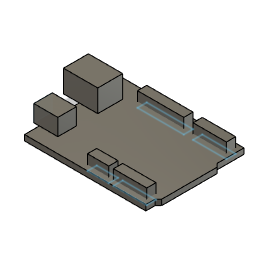
Arduino v3 (Autodesk Fusion 360 design; units mm, degrees)
Autodesk Fusion 360 part; units mm, degrees
sketch "Sketch1" plane through (0, 0, 0) normal (0, 1, 0) x (1, 0, 0)
  line L0 (0, 0) -> (65.5, 0)
  line L1 (65.5, 0) -> (65.5, -53)
  line L2 (65.5, -53) -> (0, -53)
  line L3 (0, -53) -> (0, 0)
  line L4 (65.5, -53) -> (65.5, -48) construction
  line L5 (65.5, -48) -> (67.2678, -46.2322)
  line L6 (65.5, -48) -> (68, -48) construction
  line L7 (67.2678, -46.2322) -> (67.2678, -16.2322)
  line L8 (67.2678, -16.2322) -> (65.5, -14.4645)
  line L9 (67.2678, -16.2322) -> (64.7678, -16.2322) construction
  dimension "d1" = 65.5
  dimension "d2" = 53
  dimension "d3" = 5
  dimension "d4" = 45
  dimension "d5" = 2.5
  dimension "d6" = 30
  dimension "d7" = 45
  dimension "d8" = 2.5
  constraint horizontal L0
  constraint vertical L1
  constraint horizontal L2
  constraint vertical L3
  constraint coincident L0.start L3.end
  constraint perpendicular L2 L4
  constraint horizontal L6
  constraint perpendicular L6 L7
  constraint horizontal L9
  measures "d1" distance of L0.start L0.end
  measures "d2" distance of L0.start L2.end
  measures "d3" distance of L1.end L4.end
  measures "d4" angle of L5 L6
  measures "d5" distance of L4.end L5.end
  measures "d6" distance of L5.end L7.end
  measures "d7" angle of L8 L9
  measures "d8" distance of L7.end L8.end
sketch "Sketch2" plane through (0, 0, 0) normal (0, 1, 0) x (1, 0, 0)
  line L0 (63, -2) -> (45, -2)
  line L1 (45, -2) -> (45, -7)
  line L2 (45, -7) -> (63, -7)
  line L3 (63, -7) -> (63, -2)
  line L4 (40, -2) -> (15, -2)
  line L5 (15, -2) -> (15, -7)
  line L6 (15, -7) -> (40, -7)
  line L7 (40, -7) -> (40, -2)
  line L8 (63, -50) -> (45, -50)
  line L9 (45, -50) -> (45, -45)
  line L10 (45, -45) -> (63, -45)
  line L11 (63, -45) -> (63, -50)
  line L12 (42.5, -45) -> (31, -45)
  line L13 (31, -45) -> (31, -50)
  line L14 (31, -50) -> (42.5, -50)
  line L15 (42.5, -50) -> (42.5, -45)
  constraint horizontal L0
  constraint vertical L1
  constraint horizontal L2
  constraint vertical L3
  constraint horizontal L4
  constraint vertical L5
  constraint horizontal L6
  constraint vertical L7
  constraint horizontal L8
  constraint vertical L9
  constraint horizontal L10
  constraint vertical L11
  constraint horizontal L12
  constraint vertical L13
  constraint horizontal L14
  constraint vertical L15
extrude "Extrude1" add sketch "Sketch1" sketch "Sketch2" along normal blind 3 of sketch 2 contours L0 L1 L2 L3 | L4 L5 L6 L7 makes body 1
sketch "Sketch3" plane through (0, 0, 0) normal (0, -1, 0) x (1, 0, 0)
  line L0 (67.2678, 46.2322) -> (65.5, 48)
  line L1 (65.5, 48) -> (65.5, 53)
  line L2 (65.5, 53) -> (0, 53)
  line L3 (0, 53) -> (0, 0)
  line L4 (0, 0) -> (65.5, 0)
  line L5 (65.5, 0) -> (65.5, 14.4645)
  line L6 (65.5, 14.4645) -> (67.2678, 16.2322)
  line L7 (67.2678, 16.2322) -> (67.2678, 46.2322)
extrude "Extrude2" add sketch "Sketch2" along normal blind 8 separate body makes body 2 at (51, 2.6667, 7) makes body 3 at (34.8333, 2.6667, 50) makes body 4 at (23.3333, 2.6667, 7) makes body 5 at (57, 2.6667, 50)
sketch "Sketch4" plane through (0, 3, 0) normal (0, 1, 0) x (-1, 0, 0)
  line L0 (-65.5, 48) -> (-67.2678, 46.2322)
  line L1 (-67.2678, 46.2322) -> (-67.2678, 16.2322)
  line L2 (-67.2678, 16.2322) -> (-65.5, 14.4645)
  line L3 (-65.5, 14.4645) -> (-65.5, 0)
  line L4 (-65.5, 0) -> (0, 0)
  line L5 (0, 0) -> (0, 53)
  line L6 (0, 53) -> (-65.5, 53)
  line L7 (-65.5, 53) -> (-65.5, 48)
  line L8 (0, 35) -> (-10, 35)
  line L9 (-10, 35) -> (-10, 45)
  line L10 (-10, 45) -> (0, 45)
  line L11 (0, 45) -> (0, 35)
  line L12 (0, 35) -> (3, 35)
  line L13 (3, 35) -> (3, 45)
  line L14 (3, 45) -> (0, 45)
  line L15 (0, 45) -> (0, 35)
  constraint horizontal L8
  constraint vertical L9
  constraint horizontal L10
  constraint vertical L11
  constraint coincident L5 L8.start
  constraint horizontal L12
  constraint vertical L13
  constraint horizontal L14
  constraint vertical L15
extrude "Extrude3" add sketch "Sketch4" along normal blind 9 contours L5 L11 L12 L13 L14 L15 | L5 L8 L9 L10 L11 L15 bodies 1
sketch "Sketch5" plane through (-3, 0, 0) normal (-1, 0, 0) x (0, 0, 1)
  line L0 (35, 3) -> (45, 3)
  line L1 (45, 3) -> (45, 12)
  line L2 (45, 12) -> (35, 12)
  line L3 (35, 12) -> (35, 3)
hole "Hole1" at (-3, 7.5, 40) direction (1, 0, 0) diameter 8 depth 10 tip angle 118 bodies 1
sketch "Sketch6" plane through (-3, 7.5, 40) normal (-1, 0, 0) x (0, 0, 1)
  circle A0 centre (0, 0) radius 1
  constraint coincident A0.centre origin
extrude "Extrude4" add sketch "Sketch6" against normal blind 11 separate body makes body 6
sketch "Sketch7" plane through (0, 3, 0) normal (0, 1, 0) x (-1, 0, 0)
  line L0 (-10, 45) -> (0, 45)
  line L1 (0, 45) -> (0, 53)
  line L2 (0, 53) -> (-65.5, 53)
  line L3 (-65.5, 53) -> (-65.5, 48)
  line L4 (-65.5, 48) -> (-67.2678, 46.2322)
  line L5 (-67.2678, 46.2322) -> (-67.2678, 16.2322)
  line L6 (-67.2678, 16.2322) -> (-65.5, 14.4645)
  line L7 (-65.5, 14.4645) -> (-65.5, 0)
  line L8 (-65.5, 0) -> (0, 0)
  line L9 (0, 0) -> (0, 35)
  line L10 (0, 35) -> (-10, 35)
  line L11 (-10, 35) -> (-10, 45)
  line L12 (-10, 10) -> (8.5084, 10)
  line L13 (8.5084, 10) -> (8.5084, 23.4625)
  line L14 (8.5084, 23.4625) -> (-10, 23.4625)
  line L15 (-10, 23.4625) -> (-10, 10)
  constraint horizontal L12
  constraint vertical L13
  constraint horizontal L14
  constraint vertical L15
extrude "Extrude5" add sketch "Sketch7" along normal blind 12 contours L9 L12 L13 L14 | L9 L12 L14 L15 bodies 1
sketch "Sketch8" plane through (-8.5084, 0, 0) normal (-1, 0, 0) x (0, 0, 1)
  line L0 (10, 3) -> (23.4625, 3)
  line L1 (23.4625, 3) -> (23.4625, 15)
  line L2 (23.4625, 15) -> (10, 15)
  line L3 (10, 15) -> (10, 3)
  line L4 (11.5, 13.5) -> (22, 13.5)
  line L5 (22, 13.5) -> (22, 6.5)
  line L6 (22, 6.5) -> (19.5, 4)
  line L7 (11.5, 6.5) -> (11.5, 13.5)
  line L8 (11.5, 6.5) -> (14, 4)
  line L9 (11.5, 6.5) -> (15.0355, 6.5) construction
  line L10 (14, 4) -> (19.5, 4)
  line L11 (13.5, 10) -> (20, 10)
  line L12 (20, 10) -> (20, 6.5)
  line L13 (20, 6.5) -> (13.5, 6.5)
  line L14 (13.5, 6.5) -> (13.5, 10)
  dimension "d22" = 45
  constraint horizontal L4
  constraint perpendicular L4 L5
  constraint perpendicular L4 L7
  constraint horizontal L9
  constraint perpendicular L7 L10
  constraint horizontal L11
  constraint vertical L12
  constraint horizontal L13
  constraint vertical L14
  measures "d22" angle of L8 L9
extrude "Extrude6" cut sketch "Sketch8" against normal blind 14 contours L4 L5 L6 L7 L8 L10 bodies 1
copy_body "Body->Comp1" bodies 1 removing the originals makes body 7 in component "Arduino"
copy_body "Body->Comp2" bodies 3 removing the originals makes body 8 in component "Component"
copy_body "Body->Comp3" bodies 2 removing the originals makes body 9 in component "Component'"
copy_body "Body->Comp4" bodies 5 removing the originals makes body 10 in component "Component''"
copy_body "Body->Comp5" bodies 4 removing the originals makes body 11 in component "Component'''"
copy_body "Body->Comp6" bodies 6 removing the originals makes body 12 in component "Component''''"
component "Arduino" placed x (1, 0, 0) y (0, 1, 0) z (0, 0, 1) at (0, 0, 0)
component "Component''''" placed x (1, 0, 0) y (0, 1, 0) z (0, 0, 1) at (0, 0, 0) in component "Arduino"
component "Component'''" placed x (1, 0, 0) y (0, 1, 0) z (0, 0, 1) at (0, 0, 0) in component "Arduino"
component "Component" placed x (1, 0, 0) y (0, 1, 0) z (0, 0, 1) at (0, 0, 0) in component "Arduino"
component "Component'" placed x (1, 0, 0) y (0, 1, 0) z (0, 0, 1) at (0, 0, 0) in component "Arduino"
component "Component''" placed x (1, 0, 0) y (0, 1, 0) z (0, 0, 1) at (0, 0, 0) in component "Arduino"
